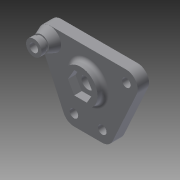
# Autodesk Inventor part: hexagon_1
Saved by Autodesk Inventor 2013 (Build 170138000, 138)
## iProperties
Created: 2013-02-11
Part Number: hexagon_1
Material: Generic
Document SubType Name: Modeling
Designer: Brad
Density: 1 g/cm^3
Author: Brad
Autodesk Inventor part; units mm, degrees
ref_plane "YZ Plane" through (0, 0, 0) normal (1, 0, 0) x (0, 1, 0)
ref_plane "XZ Plane" through (0, 0, 0) normal (0, 1, 0) x (-1, 0, 0)
ref_plane "XY Plane" through (0, 0, 0) normal (0, 0, 1) x (1, 0, 0)
sketch "Sketch1" plane through (0, 0, 0) normal (0, 0, 1) x (1, 0, 0)
  circle A0 centre (0, 0) radius 3.5
  line L0 (0, 0) -> (7.5, 0)
  line L1 (0, 0) -> (-7.5, 0)
  line L2 (7.5, 0) -> (7.5, -18.1083)
  line L3 (-7.5, 0) -> (-7.5, -18.1083)
  circle A1 centre (7.5, -18.1083) radius 2.25
  circle A2 centre (-7.5, -18.1083) radius 2.25
  circle A3 centre (0, 0) radius 22.5
  line L4 (0, 0) -> (20.25, 0)
  line L5 (20.25, 0) -> (20.25, 9.8075)
  line L6 (0, 0) -> (-20.25, 0)
  line L7 (-20.25, 0) -> (-20.25, 9.8075)
  circle A4 centre (20.25, 9.8075) radius 2.25
  circle A5 centre (-20.25, 9.8075) radius 2.25
  line L8 (-20.25, 9.8075) -> (20.25, 9.8075)
  line L9 (20.25, 9.8075) -> (7.5, -18.1083)
  line L10 (7.5, -18.1083) -> (-7.5, -18.1083)
  line L11 (-7.5, -18.1083) -> (-20.25, 9.8075)
  line L12 (-20.25, 15.8075) -> (20.25, 15.8075)
  line L13 (25.7077, 7.3148) -> (12.9577, -20.601)
  line L14 (7.5, -24.1083) -> (-7.5, -24.1083)
  line L15 (-12.9577, -20.601) -> (-25.7077, 7.3148)
  circle A6 centre (-20.25, 9.8075) radius 6
  circle A7 centre (20.25, 9.8075) radius 6
  circle A8 centre (7.5, -18.1083) radius 6
  arc A9 (-13.499, -18.0007) -> (-7.5, -24.1083) centre (-7.5, -18.1083) ccw
  arc A10 (-7.5, -18.1083) -> (7.5, -18.1083) centre (0, 0) ccw
  dimension "d0" = 7
  dimension "d1" = 7.5
  dimension "d2" = 7.5
  dimension "d4" = 4.5
  dimension "d5" = 4.5
  dimension "d6" = 45
  dimension "d7" = 20.25
  dimension "d8" = 20.25
  dimension "d9" = 4.5
  dimension "d10" = 4.5
  dimension "d11" = 6
  dimension "d27" = 12
  dimension "d28" = 6
  dimension "d29" = 12
  dimension "d30" = 12
  constraints: 32 end point, 14 point on circle, 11 centre point, 9 coincident, 4 perpendicular, 4 tangent, 2 equal length, 1 horizontal, 1 point on line
  measures "d0" diameter of A0
  measures "d1" distance of L0.start L0.end
  measures "d2" distance of L0.start L1.end
  measures "d4" diameter of A1
  measures "d5" diameter of A2
  measures "d6" diameter of A3
  measures "d7" distance of L4.start L4.end
  measures "d8" distance of L4.start L6.end
  measures "d9" diameter of A4
  measures "d10" diameter of A5
  measures "d11" distance between parallel lines of L8 L12
  measures "d27" diameter of A8
  measures "d28" radius of A9
  measures "d29" diameter of A6
  measures "d30" diameter of A7
extrude "Extrusion1" add sketch "Sketch1" along normal blind 6 contours L0 L2 A8 L10 A2 L3 L1 A0 | A0 L1 L6 L11 A6 L8 A7 L9 L4 L0 | L4 L9 A8 L2 | L3 A2 L11 L6 | A8 L9 A1 L2 | L2 A1 L10 A8 | L9 A7 L5 L4 | L4 L5 A7 A3 L13 A8 L9 | L11 A2 A10 A8 A3 L15 A6 L7 L6 | L6 L7 A6 L11 | A8 A3 A10 A1 L9 | A8 A10 A2 L10 | L10 A1 A10 A8 | A7 L8 A4 L9 | L9 A4 L5 A7 | A6 L7 A5 L11 | L11 A5 L8 A6 | A8 A3 | A3 L13 A8 | L5 A4 A3 A7 | A7 A3 A4 L8 | L8 A6 A3 L12 A7 | A6 A3 A5 L7 | L8 A5 A3 A6 | A8 L14 A9 A3 | A7 L13 A3 | A3 A4 A7 | A3 L12 A7 | A6 A3 A5 | A3 L15 A6 | A6 L12 A3 | A9 L15 A3
sketch "Sketch2" plane through (0, 0, 0) normal (0, 0, -1) x (-1, 0, 0)
  circle A0 centre (0, 0) radius 3.5 projected
  circle A1 centre (0, 0) radius 6.5
  circle A2 centre (0, 0) radius 3.5
  dimension "d14" = 13
  constraints: 2 centre point, 2 coincident, 1 concentric
  measures "d14" diameter of A1
extrude "Extrusion2" add sketch "Sketch2" along normal blind 4.5
fillet "Fillet1" radius 3 1 edges at (6.5, 0, 0)
sketch "Sketch3" plane through (0, 0, 6) normal (0, 0, 1) x (1, 0, 0)
  circle A0 centre (-20.25, 9.8075) radius 2.25 projected
  arc A1 (-20.25, 15.8075) -> (-25.7077, 7.3148) centre (-20.25, 9.8075) ccw projected
  circle A2 centre (-20.25, 9.8075) radius 4.125
  circle A3 centre (-20.25, 9.8075) radius 2.25
  dimension "d18" = 8.25
  dimension "d36" = 4.5
  constraints: 2 centre point, 2 coincident, 1 concentric
  measures "d18" diameter of A2
  measures "d36" diameter of A0
extrude "Extrusion3" add sketch "Sketch3" along normal blind 4.5
sketch "Sketch4" plane through (-20.25, 9.8075, 10.5) normal (0, 0, 1) x (1, 0, 0)
  circle A0 centre (0, 0) radius 2.25 projected
  circle A1 centre (0, 0) radius 4.125 projected
  circle A2 centre (0, 0) radius 3.5
  circle A3 centre (0, 0) radius 2.25
  point P0 (20.25, -9.8075)
  dimension "d21" = 7
  constraints: 2 centre point, 2 coincident, 1 concentric
  measures "d21" diameter of A2
extrude "Extrusion4" add sketch "Sketch4" along normal blind 1.5 contours A2
sketch "Sketch5" plane through (-20.25, 9.8075, 12) normal (0, 0, 1) x (1, 0, 0)
  circle A0 centre (0, 0) radius 2.25 projected
  circle A1 centre (0, 0) radius 3.5 projected
  circle A2 centre (0, 0) radius 4.125
  circle A3 centre (0, 0) radius 2.25
  point P0 (20.25, -9.8075)
  dimension "d24" = 8.25
  constraints: 2 centre point, 2 coincident, 1 concentric
  measures "d24" diameter of A2
extrude "Extrusion5" add sketch "Sketch5" along normal blind 2.5 contours A1 | A2
sketch "Sketch6" plane through (0, 0, 6) normal (0, 0, 1) x (1, 0, 0)
  circle A0 centre (0, 0) radius 3.5 projected
  line L0 (6.6973, 0) -> (3.3486, -5.8)
  line L1 (3.3486, -5.8) -> (-3.3486, -5.8)
  line L2 (-3.3486, -5.8) -> (-6.6973, 0)
  line L3 (-6.6973, 0) -> (-3.3486, 5.8)
  line L4 (-3.3486, 5.8) -> (3.3486, 5.8)
  line L5 (3.3486, 5.8) -> (6.6973, 0)
  circle A1 centre (0, 0) radius 9
  dimension "d31" = 11.6
  dimension "d32" = 18
  constraints: 12 end point, 2 coincident, 1 centre point, 13 other
  measures "d31" distance between parallel lines of L1 L4
  measures "d32" diameter of A1
extrude "Extrusion6" add sketch "Sketch6" along normal blind 4 contours A1
fillet "Fillet2" radius 2 1 edges at (-9, 0, 6)
draft "FaceDraft1" angle 22 pull direction (0, 0, 1) faces at (-16.1384, 9.4756, 9) fixed edges at (-24.375, 9.8075, 10.5)
body "Solid1"
